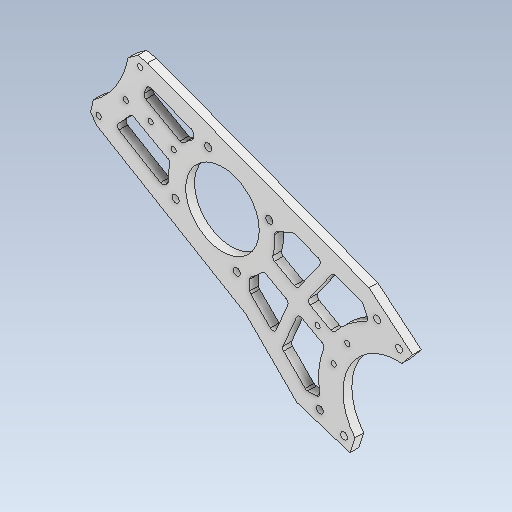
# Autodesk Inventor part: motor_r_1
Saved by Autodesk Inventor 2020 (Build 240168000, 168)
## iProperties
Created: 2020-08-12
Part Number: motor_r_1
Material: ABS Plastic
Document SubType Name: Modeling
Designer: psrobotics
Density: 1.06 g/cm^3
Appearance: Smooth - White
Author: psrobotics
Autodesk Inventor part; units mm, degrees
ref_plane "YZ Plane" through (0, 0, 0) normal (1, 0, 0) x (0, 1, 0)
ref_plane "XZ Plane" through (0, 0, 0) normal (0, 1, 0) x (-1, 0, 0)
ref_plane "XY Plane" through (0, 0, 0) normal (0, 0, 1) x (1, 0, 0)
sketch "Sketch1" plane through (0, 0, 0) normal (0, 0, 1) x (1, 0, 0)
  circle A0 centre (-61.1849, 56.2101) radius 2 projected
  circle A1 centre (-79.1833, 55.9721) radius 2 projected
  circle A2 centre (-87.9764, 40.2661) radius 2 projected
  circle A3 centre (-78.7712, 24.7979) radius 2 projected
  circle A4 centre (-60.7727, 25.0359) radius 2 projected
  circle A5 centre (-51.9796, 40.742) radius 2 projected
  circle A6 centre (39.2427, 1.4435) radius 2.05 projected
  circle A7 centre (33.5273, 15.312) radius 2.05 projected
  circle A8 centre (27.8118, 29.1804) radius 2.05 projected
  line L0 (-22.6947, 30.3679) -> (-27.7397, 36.0115) projected
  arc A9 (-27.2107, 40.4775) -> (-27.7397, 36.0115) centre (-25.5031, 38.0109) ccw projected
  arc A10 (-20.7425, 44.2388) -> (-27.2107, 40.4775) centre (-0.1733, 1.4234) ccw projected
  arc A11 (-16.6578, 42.6485) -> (-20.7425, 44.2388) centre (-19.4434, 41.5346) ccw projected
  line L1 (-16.6578, 42.6485) -> (-13.8655, 35.6655) projected
  arc A12 (-15.3151, 31.8656) -> (-13.8655, 35.6655) centre (-16.6511, 34.5516) ccw projected
  arc A13 (-15.3151, 31.8656) -> (-18.8133, 29.8584) centre (-0.1733, 1.4234) ccw projected
  arc A14 (-22.6947, 30.3679) -> (-18.8133, 29.8584) centre (-20.4581, 32.3673) ccw projected
  line L2 (4.9218, -40.8928) -> (6.6144, -39.5468) projected
  arc A15 (9.7386, -40.4282) -> (6.6144, -39.5468) centre (7.8592, -41.1122) ccw projected
  line L3 (9.7386, -40.4282) -> (10.4367, -42.3462) projected
  arc A16 (8.0919, -44.9753) -> (10.4367, -42.3462) centre (8.5573, -43.0302) ccw projected
  line L4 (8.0919, -44.9753) -> (5.7012, -44.4033) projected
  arc A17 (4.9218, -40.8928) -> (5.7012, -44.4033) centre (6.1666, -42.4582) ccw projected
  line L5 (-46.4911, 13.9051) -> (-45.8812, 17.2926) projected
  arc A18 (-42.9676, 18.7008) -> (-45.8812, 17.2926) centre (-43.9129, 16.9383) ccw projected
  line L6 (-42.9676, 18.7008) -> (-40.9403, 17.6135) projected
  arc A19 (-40.5709, 14.3438) -> (-40.9403, 17.6135) centre (-41.8856, 15.851) ccw projected
  line L7 (-40.5709, 14.3438) -> (-43.208, 12.0435) projected
  arc A20 (-46.4911, 13.9051) -> (-43.208, 12.0435) centre (-44.5227, 13.5507) ccw projected
  arc A21 (20.902, 43.992) -> (13.9559, 46.7733) centre (-0.1733, 1.4234) ccw projected
  arc A22 (22.1637, 39.7941) -> (20.902, 43.992) centre (19.571, 41.3034) ccw projected
  line L8 (22.1637, 39.7941) -> (18.3801, 33.2946) projected
  arc A23 (14.4933, 32.0974) -> (18.3801, 33.2946) centre (15.7874, 34.8039) ccw projected
  arc A24 (14.4933, 32.0974) -> (10.7578, 33.6183) centre (-0.1733, 1.4234) ccw projected
  arc A25 (8.7698, 36.9905) -> (10.7578, 33.6183) centre (11.7223, 36.459) ccw projected
  line L9 (8.7698, 36.9905) -> (10.111, 44.4407) projected
  arc A26 (13.9559, 46.7733) -> (10.111, 44.4407) centre (13.0635, 43.9091) ccw projected
  line L10 (15.012, -40.2978) -> (12.4398, -33.2308) projected
  arc A27 (14.0077, -29.4781) -> (12.4398, -33.2308) centre (15.2589, -32.2047) ccw projected
  arc A28 (14.0077, -29.4781) -> (21.8399, -24.4884) centre (-0.1733, 1.4234) ccw projected
  arc A29 (25.9036, -24.6534) -> (21.8399, -24.4884) centre (23.7822, -26.7747) ccw projected
  line L11 (25.9036, -24.6534) -> (31.2214, -29.9713) projected
  arc A30 (31.0736, -34.3521) -> (31.2214, -29.9713) centre (29.1001, -32.0926) ccw projected
  arc A31 (19.0449, -42.0152) -> (31.0736, -34.3521) centre (-0.1733, 1.4234) ccw projected
  arc A32 (15.012, -40.2978) -> (19.0449, -42.0152) centre (17.8311, -39.2717) ccw projected
  line L12 (-31.4674, 32.6792) -> (-26.4223, 27.0356) projected
  arc A33 (-26.3493, 23.1217) -> (-26.4223, 27.0356) centre (-28.659, 25.0362) ccw projected
  arc A34 (-26.3493, 23.1217) -> (-28.7345, 19.8693) centre (-0.1733, 1.4234) ccw projected
  arc A35 (-32.6725, 18.8531) -> (-28.7345, 19.8693) centre (-31.2547, 21.4969) ccw projected
  line L13 (-32.6725, 18.8531) -> (-39.3001, 22.4076) projected
  arc A36 (-40.4244, 26.6443) -> (-39.3001, 22.4076) centre (-37.8823, 25.0514) ccw projected
  arc A37 (-35.9645, 32.6522) -> (-40.4244, 26.6443) centre (-0.1733, 1.4234) ccw projected
  arc A38 (-31.4674, 32.6792) -> (-35.9645, 32.6522) centre (-33.704, 30.6798) ccw projected
  line L14 (37.0627, -22.7579) -> (30.7554, -18.6619) projected
  arc A39 (29.7491, -14.7214) -> (30.7554, -18.6619) centre (32.3893, -16.1459) ccw projected
  arc A40 (29.7491, -14.7214) -> (31.8466, -10.0103) centre (-0.1733, 1.4234) ccw projected
  arc A41 (35.4483, -8.1214) -> (31.8466, -10.0103) centre (34.6719, -11.0192) ccw projected
  line L15 (35.4483, -8.1214) -> (42.7127, -10.0678) projected
  arc A42 (44.775, -13.9357) -> (42.7127, -10.0678) centre (41.9362, -12.9656) ccw projected
  arc A43 (41.317, -21.7025) -> (44.775, -13.9357) centre (-0.1733, 1.4234) ccw projected
  arc A44 (37.0627, -22.7579) -> (41.317, -21.7025) centre (38.6966, -20.2419) ccw projected
  line L16 (5.1901, 45.3265) -> (3.8489, 37.8764) projected
  arc A45 (0.8096, 35.4092) -> (3.8489, 37.8764) centre (0.8963, 38.4079) ccw projected
  arc A46 (0.8096, 35.4092) -> (-3.2217, 35.2865) centre (-0.1733, 1.4234) ccw projected
  arc A47 (-6.447, 37.764) -> (-3.2217, 35.2865) centre (-3.4907, 38.2744) ccw projected
  line L17 (-6.447, 37.764) -> (-7.7264, 45.175) projected
  arc A48 (-5.08, 48.6693) -> (-7.7264, 45.175) centre (-4.7701, 45.6853) ccw projected
  arc A49 (2.4, 48.8536) -> (-5.08, 48.6693) centre (-0.1733, 1.4234) ccw projected
  arc A50 (5.1901, 45.3265) -> (2.4, 48.8536) centre (2.2375, 45.858) ccw projected
  line L18 (1.7065, -37.0615) -> (-5.4722, -42.7701) projected
  line L19 (-5.4722, -42.7701) -> (-0.1588, -48.8615) projected
  arc A51 (0.3036, -49.8289) -> (-0.1588, -48.8615) centre (-1.666, -50.1762) ccw projected
  line L20 (0.3036, -49.8289) -> (1.5962, -57.1593) projected
  line L21 (1.5962, -57.1593) -> (13.8376, -55.0009) projected
  line L22 (13.8376, -55.0009) -> (13.4343, -52.7138) projected
  arc A52 (14.8476, -50.4454) -> (13.4343, -52.7138) centre (15.4039, -52.3665) ccw projected
  arc A53 (14.8476, -50.4454) -> (24.4955, -46.6125) centre (-0.1733, 1.4234) ccw projected
  arc A54 (27.0802, -47.2926) -> (24.4955, -46.6125) centre (25.4092, -48.3917) ccw projected
  line L23 (27.0802, -47.2926) -> (28.3563, -49.2329) projected
  line L24 (28.3563, -49.2329) -> (35.0402, -44.8369) projected
  line L25 (35.0402, -44.8369) -> (33.7641, -42.8966) projected
  arc A55 (34.1633, -40.2539) -> (33.7641, -42.8966) centre (35.435, -41.7975) ccw projected
  arc A56 (34.1633, -40.2539) -> (41.5041, -32.9132) centre (-0.1733, 1.4234) ccw projected
  arc A57 (44.1467, -32.5139) -> (41.5041, -32.9132) centre (43.0477, -34.1849) ccw projected
  line L26 (44.1467, -32.5139) -> (46.087, -33.7901) projected
  line L27 (46.087, -33.7901) -> (50.4831, -27.1062) projected
  line L28 (50.4831, -27.1062) -> (48.5428, -25.83) projected
  arc A58 (47.8627, -23.2454) -> (48.5428, -25.83) centre (49.6418, -24.159) ccw projected
  arc A59 (47.8627, -23.2454) -> (51.6956, -13.5974) centre (-0.1733, 1.4234) ccw projected
  arc A60 (53.9639, -12.1842) -> (51.6956, -13.5974) centre (53.6166, -14.1538) ccw projected
  line L29 (53.9639, -12.1842) -> (56.251, -12.5874) projected
  line L30 (56.251, -12.5874) -> (57.764, -4.0066) projected
  line L31 (57.764, -4.0066) -> (50.7504, -2.7699) projected
  arc A61 (49.2479, -1.5605) -> (50.7504, -2.7699) centre (51.0977, -0.8002) ccw projected
  line L32 (49.2479, -1.5605) -> (34.2938, 34.8242) projected
  arc A62 (34.7161, 36.9851) -> (34.2938, 34.8242) centre (36.1437, 35.5844) ccw projected
  line L33 (34.7161, 36.9851) -> (37.6444, 39.9698) projected
  line L34 (37.6444, 39.9698) -> (40.1908, 42.9826) projected
  line L35 (40.1908, 42.9826) -> (34.0809, 48.1469) projected
  line L36 (34.0809, 48.1469) -> (33.2883, 47.209) projected
  arc A63 (29.3565, 46.6339) -> (33.2883, 47.209) centre (30.9971, 49.1456) ccw projected
  arc A64 (29.3565, 46.6339) -> (19.0204, 51.8972) centre (-0.1733, 1.4234) ccw projected
  arc A65 (17.5237, 53.1421) -> (19.0204, 51.8972) centre (20.0867, 54.7013) ccw projected
  line L37 (17.5237, 53.1421) -> (1.2772, 56.0668) projected
  arc A66 (-0.5596, 55.422) -> (1.2772, 56.0668) centre (-0.5811, 58.4219) ccw projected
  arc A67 (-0.5596, 55.422) -> (-12.0824, 54.0938) centre (-0.1733, 1.4234) ccw projected
  arc A68 (-15.5667, 56.004) -> (-12.0824, 54.0938) centre (-12.744, 57.0199) ccw projected
  line L38 (-15.5667, 56.004) -> (-15.9826, 57.1593) projected
  line L39 (-15.9826, 57.1593) -> (-66.6416, 64.271) projected
  arc A69 (-66.6416, 64.271) -> (-80.5887, 18.977) centre (-69.978, 40.504) ccw projected
  line L40 (-80.5887, 18.977) -> (-57.764, 7.7267) projected
  line L41 (-57.764, 7.7267) -> (-53.8816, 7.0278) projected
  line L42 (-53.8816, 7.0278) -> (-49.1938, 6.5386) projected
  arc A70 (-47.8942, 5.8641) -> (-49.1938, 6.5386) centre (-49.4014, 4.5494) ccw projected
  line L43 (-47.8942, 5.8641) -> (-45.6437, 3.2841) projected
  line L44 (-45.6437, 3.2841) -> (-37.685, 10.2263) projected
  arc A71 (-31.0721, 6.849) -> (-37.685, 10.2263) centre (-35.0556, 7.2119) ccw projected
  line L45 (-31.0721, 6.849) -> (-32.7441, -11.5046) projected
  line L46 (-32.7441, -11.5046) -> (-18.0587, -28.3404) projected
  line L47 (-18.0587, -28.3404) -> (-0.4203, -29.9472) projected
  arc A72 (1.7065, -37.0615) -> (-0.4203, -29.9472) centre (-0.7832, -33.9307) ccw projected
  line L48 (-19.335, 18.2488) -> (-14.2914, 9.8007) projected
  arc A73 (-15.0846, 8.2903) -> (-14.2914, 9.8007) centre (-15.1501, 9.2881) ccw projected
  line L49 (-15.0846, 8.2903) -> (-24.9026, 7.6464) projected
  arc A74 (-26.4331, 9.5885) -> (-24.9026, 7.6464) centre (-25.0008, 9.1432) ccw projected
  arc A75 (-21.8027, 18.4062) -> (-26.4331, 9.5885) centre (-0.1733, 1.4234) ccw projected
  arc A76 (-19.335, 18.2488) -> (-21.8027, 18.4062) centre (-20.6229, 17.4799) ccw projected
  line L50 (-25.62, -0.2287) -> (-16.08, -2.636) projected
  arc A77 (-15.5728, -4.2649) -> (-16.08, -2.636) centre (-16.3246, -3.6056) ccw projected
  line L51 (-15.5728, -4.2649) -> (-22.0599, -11.6626) projected
  arc A78 (-24.5154, -11.3715) -> (-22.0599, -11.6626) centre (-23.1877, -10.6736) ccw projected
  arc A79 (-27.4763, -1.8623) -> (-24.5154, -11.3715) centre (-0.1733, 1.4234) ccw projected
  arc A80 (-25.62, -0.2287) -> (-27.4763, -1.8623) centre (-25.987, -1.6831) ccw projected
  line L52 (-16.9986, -17.7383) -> (-8.5506, -12.6948) projected
  arc A81 (-7.0401, -13.488) -> (-8.5506, -12.6948) centre (-8.038, -13.5534) ccw projected
  line L53 (-7.0401, -13.488) -> (-6.3962, -23.3059) projected
  arc A82 (-8.3384, -24.8365) -> (-6.3962, -23.3059) centre (-7.893, -23.4041) ccw projected
  arc A83 (-17.1561, -20.2061) -> (-8.3384, -24.8365) centre (-0.1733, 1.4234) ccw projected
  arc A84 (-16.9986, -17.7383) -> (-17.1561, -20.2061) centre (-16.2297, -19.0263) ccw projected
  line L54 (1.4788, -24.0233) -> (3.8861, -14.4833) projected
  arc A85 (5.5151, -13.9761) -> (3.8861, -14.4833) centre (4.8558, -14.728) ccw projected
  line L55 (5.5151, -13.9761) -> (12.9127, -20.4632) projected
  arc A86 (12.6216, -22.9188) -> (12.9127, -20.4632) centre (11.9237, -21.591) ccw projected
  arc A87 (3.1124, -25.8796) -> (12.6216, -22.9188) centre (-0.1733, 1.4234) ccw projected
  arc A88 (1.4788, -24.0233) -> (3.1124, -25.8796) centre (2.9332, -24.3904) ccw projected
  line L56 (18.9885, -15.402) -> (13.9449, -6.9539) projected
  arc A89 (14.7381, -5.4435) -> (13.9449, -6.9539) centre (14.8035, -6.4413) ccw projected
  line L57 (14.7381, -5.4435) -> (24.5561, -4.7996) projected
  arc A90 (26.0866, -6.7418) -> (24.5561, -4.7996) centre (24.6543, -6.2964) ccw projected
  arc A91 (21.4562, -15.5594) -> (26.0866, -6.7418) centre (-0.1733, 1.4234) ccw projected
  arc A92 (18.9885, -15.402) -> (21.4562, -15.5594) centre (20.2764, -14.6331) ccw projected
  line L58 (25.2735, 3.0755) -> (15.7335, 5.4828) projected
  arc A93 (15.2263, 7.1117) -> (15.7335, 5.4828) centre (15.9781, 6.4524) ccw projected
  line L59 (15.2263, 7.1117) -> (21.7134, 14.5094) projected
  arc A94 (24.1689, 14.2183) -> (21.7134, 14.5094) centre (22.8412, 13.5204) ccw projected
  arc A95 (27.1298, 4.7091) -> (24.1689, 14.2183) centre (-0.1733, 1.4234) ccw projected
  arc A96 (25.2735, 3.0755) -> (27.1298, 4.7091) centre (25.6405, 4.5299) ccw projected
  line L60 (16.6521, 20.5851) -> (8.2041, 15.5416) projected
  arc A97 (6.6936, 16.3348) -> (8.2041, 15.5416) centre (7.6915, 16.4002) ccw projected
  line L61 (6.6936, 16.3348) -> (6.0497, 26.1527) projected
  arc A98 (7.9919, 27.6833) -> (6.0497, 26.1527) centre (7.5465, 26.2509) ccw projected
  arc A99 (16.8096, 23.0529) -> (7.9919, 27.6833) centre (-0.1733, 1.4234) ccw projected
  arc A100 (16.6521, 20.5851) -> (16.8096, 23.0529) centre (15.8832, 21.8731) ccw projected
  line L62 (-1.8253, 26.8701) -> (-4.2326, 17.3301) projected
  arc A101 (-5.8616, 16.8229) -> (-4.2326, 17.3301) centre (-5.2023, 17.5748) ccw projected
  line L63 (-5.8616, 16.8229) -> (-13.2592, 23.31) projected
  arc A102 (-12.9681, 25.7656) -> (-13.2592, 23.31) centre (-12.2702, 24.4378) ccw projected
  arc A103 (-3.4589, 28.7264) -> (-12.9681, 25.7656) centre (-0.1733, 1.4234) ccw projected
  arc A104 (-1.8253, 26.8701) -> (-3.4589, 28.7264) centre (-3.2797, 27.2372) ccw projected
  circle A105 centre (10.0674, -10.8701) radius 2 projected
  circle A106 centre (-10.4139, 13.7169) radius 2 projected
  circle A107 centre (-15.1114, 2.7842) radius 1.5 projected
  circle A108 centre (14.7649, 0.0626) radius 1.5 projected
  circle A109 centre (-1.5341, -13.5147) radius 1.5 projected
  circle A110 centre (1.1876, 16.3615) radius 1.5 projected
  circle A111 centre (-12.4667, -8.8173) radius 2 projected
  circle A112 centre (12.1202, 11.664) radius 2 projected
  circle A113 centre (-0.1733, 1.4234) radius 12 projected
  circle A114 centre (-18.3916, 52.0411) radius 1.55 projected
  circle A115 centre (53.4988, -8.0404) radius 1.55 projected
  circle A116 centre (29.775, -44.1107) radius 1.55 projected
  circle A117 centre (9.2906, -52.2486) radius 1.55 projected
  circle A118 centre (45.3608, -28.5248) radius 1.55 projected
  circle A119 centre (34.5538, 42.5098) radius 1.55 projected
  circle A120 centre (-53.1186, 10.9547) radius 1.55 projected
  circle A121 centre (200.5155, -110.9334) radius 35 projected
  line L64 (28.3563, -49.2329) -> (182.6199, -141.0124)
  line L65 (57.764, -4.0066) -> (215.5932, -79.3476)
  circle A122 centre (-0.1733, 1.4234) radius 47.5
  line L66 (28.3563, -49.2329) -> (22.4938, -40.3193)
  line L67 (57.764, -4.0066) -> (47.1927, -2.1425)
  point P0 (0, 0)
  point P1 (44.775, -13.9357)
  point P2 (41.317, -21.7025)
  constraints: 8 end point, 4 point on circle, 2 collinear, 2 tangent, 1 centre point, 1 coincident, 1 concentric
extrude "Extrusion1" add sketch "Sketch1" along normal blind 5 contours A31 A122 A43 L67 L31 L30 L29 A60 A59 A58 L28 L27 L26 A57 A56 A55 L25 L24 L23 L66 | L65 A121 L64 L24 L25 A55 A56 A57 L26 L27 L28 A58 A59 A60 L29 L30
sketch "Sketch2" plane through (0, 0, 5) normal (0, 0, 1) x (1, 0, 0)
  circle A0 centre (100.6074, -54.9992) radius 17.5 projected
  circle A1 centre (100.6074, -54.9992) radius 21
  point P0 (0, 0)
  dimension "d5" = 42
  constraints: 1 centre point, 1 coincident
  measures "d5" diameter of A1
extrude "Extrusion2" cut sketch "Sketch2" against normal blind 5 contours A0 | A1
sketch "Sketch3" plane through (0, 0, 5) normal (0, 0, 1) x (1, 0, 0)
  circle A0 centre (156.3377, -126.3623) radius 2 projected
  circle A1 centre (170.0821, -132.37) radius 2 projected
  line L0 (189.8622, -144.2727) -> (191.6885, -138.5574) projected
  arc A2 (185.6877, -135.856) -> (191.6885, -138.5574) centre (200.5155, -110.9334) ccw projected
  line L1 (151.3117, -115.4039) -> (185.6877, -135.856) projected
  line L2 (143.0379, -129.3104) -> (151.3117, -115.4039) projected
  line L3 (189.8622, -144.2727) -> (143.0379, -129.3104) projected
  circle A3 centre (201.5033, -73.4985) radius 2 projected
  circle A4 centre (188.9781, -65.2451) radius 2 projected
  line L4 (184.3455, -51.955) -> (222.8987, -84.0263) projected
  line L5 (176.9104, -67.5306) -> (184.3455, -51.955) projected
  line L6 (213.0084, -84.7623) -> (176.9104, -67.5306) projected
  arc A5 (219.0616, -88.6389) -> (213.0084, -84.7623) centre (200.5155, -110.9334) ccw projected
  line L7 (219.0616, -88.6389) -> (222.8987, -84.0263) projected
  arc A6 (215.5932, -79.3476) -> (182.6199, -141.0124) centre (200.5155, -110.9334) ccw projected
  line L8 (200.5155, -110.9334) -> (182.1469, -141.8073)
  line L9 (200.5155, -110.9334) -> (216.071, -78.3466)
  point P0 (0, 0)
  constraints: 4 end point, 4 point on line
extrude "Extrusion3" add sketch "Sketch3" against normal blind 5 contours A0 | A1 | L3 L2 L1 A6 L8 | L8 A6 L1 | A6 L9 L6 | L6 L5 L4 L9 A6 | A3 | A4
thicken "Thicken1" operation add thickness 4 both sides no extend neighbours yes toward (0.637995, -0.7700405, 0) faces at (178.1856, -83.982, 3.3333)
sketch "Sketch4" plane through (0, 0, 5) normal (0, 0, 1) x (1, 0, 0)
  circle A0 centre (53.4988, -8.0404) radius 1.55 projected
  circle A1 centre (29.775, -44.1107) radius 1.55 projected
  circle A2 centre (45.3608, -28.5248) radius 1.55 projected
  circle A3 centre (100.6074, -54.9992) radius 21 projected
  line L0 (213.0084, -84.7623) -> (216.071, -78.3466) projected
  line L1 (216.071, -78.3466) -> (184.3455, -51.955) projected
  line L2 (184.3455, -51.955) -> (179.4951, -62.1159) projected
  line L3 (179.4951, -62.1159) -> (57.764, -4.0066) projected
  line L4 (57.764, -4.0066) -> (47.1927, -2.1425) projected
  arc A4 (22.4938, -40.3193) -> (47.1927, -2.1425) centre (-0.1733, 1.4234) ccw projected
  line L5 (22.4938, -40.3193) -> (28.3563, -49.2329) projected
  line L6 (28.3563, -49.2329) -> (148.2438, -120.5603) projected
  line L7 (148.2438, -120.5603) -> (143.0379, -129.3104) projected
  line L8 (143.0379, -129.3104) -> (182.1469, -141.8073) projected
  line L9 (182.1469, -141.8073) -> (185.6877, -135.856) projected
  line L10 (185.6877, -135.856) -> (176.2734, -130.255) projected
  arc A5 (203.1226, -80.0432) -> (176.2734, -130.255) centre (200.5155, -110.9334) ccw projected
  line L11 (203.1226, -80.0432) -> (213.0084, -84.7623) projected
  line L12 (179.4951, -62.1159) -> (57.764, -4.0066) projected
  line L13 (148.2438, -120.5603) -> (143.0379, -129.3104) projected
  line L14 (148.2438, -120.5603) -> (113.8678, -100.1082)
  line L15 (28.3563, -49.2329) -> (148.2438, -120.5603) projected
  line L16 (143.0379, -129.3104) -> (182.1469, -141.8073) projected
  line L17 (113.8678, -100.1082) -> (143.0379, -129.3104)
  line L18 (184.3455, -51.955) -> (57.764, -4.0066)
  point P0 (0, 0)
  dimension "d13" = 40
  constraints: 6 end point, 1 point on line
  measures "d13" distance of L6.end L14.end
extrude "Extrusion4" add sketch "Sketch4" against normal blind 5 contours L2 L3 L18 | L17 L6 L7
sketch "Sketch5" plane through (0, 0, 5) normal (0, 0, 1) x (1, 0, 0)
  circle A0 centre (188.9781, -65.2451) radius 2 projected
  circle A1 centre (201.5033, -73.4985) radius 2 projected
  circle A2 centre (156.3377, -126.3623) radius 2 projected
  circle A3 centre (170.0821, -132.37) radius 2 projected
  point P0 (0, 0)
extrude "Extrusion5" cut sketch "Sketch5" against normal blind 10
sketch "Sketch6" plane through (0, 0, 0) normal (0, 0, -1) x (-1, 0, 0)
  circle A0 centre (-156.3377, -126.3623) radius 2 projected
  circle A1 centre (-201.5033, -73.4985) radius 2 projected
  circle A2 centre (-170.0821, -132.37) radius 2 projected
  circle A3 centre (-188.9781, -65.2451) radius 2 projected
  arc A4 (-176.2734, -130.255) -> (-203.1226, -80.0432) centre (-200.5155, -110.9334) ccw projected
  line L0 (-176.2734, -130.255) -> (-185.6877, -135.856) projected
  line L1 (-185.6877, -135.856) -> (-182.1469, -141.8073) projected
  line L2 (-182.1469, -141.8073) -> (-143.0379, -129.3104) projected
  line L3 (-143.0379, -129.3104) -> (-113.8678, -100.1082) projected
  line L4 (-28.3563, -49.2329) -> (-113.8678, -100.1082) projected
  line L5 (-22.4938, -40.3193) -> (-28.3563, -49.2329) projected
  arc A5 (-47.1927, -2.1425) -> (-22.4938, -40.3193) centre (0.1733, 1.4234) ccw projected
  line L6 (-57.764, -4.0066) -> (-47.1927, -2.1425) projected
  line L7 (-57.764, -4.0066) -> (-184.3455, -51.955) projected
  line L8 (-184.3455, -51.955) -> (-216.071, -78.3466) projected
  line L9 (-216.071, -78.3466) -> (-213.0084, -84.7623) projected
  line L10 (-213.0084, -84.7623) -> (-203.1226, -80.0432) projected
  circle A6 centre (-100.6074, -54.9992) radius 21 projected
  circle A7 centre (-45.3608, -28.5248) radius 1.55 projected
  circle A8 centre (-29.775, -44.1107) radius 1.55 projected
  circle A9 centre (-53.4988, -8.0404) radius 1.55 projected
  arc A10 (-176.2734, -130.255) -> (-203.1226, -80.0432) centre (-200.5155, -110.9334) ccw projected
  line L11 (-203.1226, -80.0432) -> (-209.2525, -72.6744)
  line L12 (-216.071, -78.3466) -> (-184.3455, -51.955) projected
  line L13 (-176.2734, -130.255) -> (-173.4681, -139.0341)
  line L14 (-143.0379, -129.3104) -> (-182.1469, -141.8073) projected
  point P0 (0, 0)
  constraints: 4 end point, 2 perpendicular, 2 point on line
extrude "Extrusion6" cut sketch "Sketch6" against normal blind 10 contours L13 L2 L1 L0 | L10 L9 L8 L11
sketch "Sketch7" plane through (0, 0, 5) normal (0, 0, 1) x (1, 0, 0)
  circle A0 centre (171.9207, -85.756) radius 2.05 projected
  circle A1 centre (164.1045, -99.7169) radius 2.05 projected
  circle A2 centre (154.9242, -85.4088) radius 2.05 projected
  circle A3 centre (72.6855, -39.367) radius 2.05 projected
  circle A4 centre (59.5971, -32.0394) radius 2.05 projected
  point P0 (0, 0)
hole "Hole1" at (59.5971, -32.0394, 5) at (72.6855, -39.367, 5) at (154.9242, -85.4088, 5) at (171.9207, -85.756, 5) at (164.1045, -99.7169, 5) direction (0, 0, -1) diameter 3 depth 8
sketch "Sketch8" plane through (0, 0, 5) normal (0, 0, 1) x (1, 0, 0)
  circle A0 centre (100.6074, -54.9992) radius 21 projected
  circle A1 centre (72.6855, -39.367) radius 1.5 projected
  circle A2 centre (72.6855, -39.367) radius 1.5 projected
  line L0 (100.6074, -54.9992) -> (72.6855, -39.367)
  line L1 (100.6074, -54.9992) -> (92.421, -28.2227)
  line L2 (100.6074, -54.9992) -> (128.6074, -54.9992) construction
  circle A3 centre (92.421, -28.2227) radius 2.05
  circle A4 centre (73.8308, -63.1856) radius 2.05
  circle A5 centre (108.7938, -81.7758) radius 2.05
  circle A6 centre (127.3839, -46.8128) radius 2.05
  point P0 (0, 0)
  dimension "d27" = 28
  dimension "d28" = 107
  dimension "d29" = 4.1
  dimension "d32" = 360
  constraints: 6 end point, 4 centre point, 1 coincident, 1 equal length, 1 horizontal, 9 other
  measures "d27" distance of L0.start L1.end
  measures "d28" angle of L2 L1
  measures "d29" diameter of A3
extrude "Extrusion7" cut sketch "Sketch8" against normal blind 10 contours A3 | A4 | A5 | A6
sketch "Sketch9" plane through (0, 0, 5) normal (0, 0, 1) x (1, 0, 0)
  arc A0 (203.1226, -80.0432) -> (176.2734, -130.255) centre (200.5155, -110.9334) ccw projected
  circle A1 centre (200.5155, -110.9334) radius 45
  circle A2 centre (100.6074, -54.9992) radius 21 projected
  circle A3 centre (100.6074, -54.9992) radius 30
  line L0 (100.6074, -54.9992) -> (200.5155, -110.9334)
  line L1 (100.6074, -54.9992) -> (200.5155, -110.9334) construction
  line L2 (97.1878, -61.1072) -> (197.0959, -117.0413)
  line L3 (203.935, -104.8255) -> (104.0269, -48.8913)
  arc A4 (104.0269, -48.8913) -> (97.1878, -61.1072) centre (100.6074, -54.9992) ccw
  arc A5 (197.0959, -117.0413) -> (203.935, -104.8255) centre (200.5155, -110.9334) ccw
  line L4 (113.8678, -100.1082) -> (143.0379, -129.3104) projected
  line L5 (111.0396, -83.127) -> (161.9072, -134.0505)
  line L6 (184.3455, -51.955) -> (57.764, -4.0066) projected
  line L7 (127.1273, -40.9744) -> (194.1952, -66.3794)
  line L8 (180.8032, -61.3066) -> (184.2573, -68.973)
  line L9 (148.4428, -120.5713) -> (156.5607, -120.5757)
  line L10 (130.3492, -51.0716) -> (141.0527, -46.2493)
  line L11 (116.2637, -80.5899) -> (116.2594, -88.3525)
  point P0 (0, 0)
  point P1 (150.5614, -82.9663)
  point P2 (158.3087, -95.326)
  point P3 (122.6421, -75.3579)
  point P4 (129.4812, -63.142)
  point P5 (165.1478, -83.1102)
  dimension "d36" = 90
  dimension "d37" = 60
  dimension "d38" = 14
  dimension "d39" = 10
  dimension "d40" = 10
  dimension "d43" = 45
  dimension "d44" = 45
  dimension "d45" = 45
  dimension "d46" = 45
  constraints: 22 end point, 12 point on circle, 4 centre point, 4 point on line, 4 tangent, 3 parallel, 2 coincident, 1 collinear, 1 midpoint
  measures "d36" diameter of A1
  measures "d37" diameter of A3
  measures "d38" diameter of A5
  measures "d39" distance between parallel lines of L4 L5
  measures "d40" distance between parallel lines of L6 L7
  measures "d43" angle of L7 L10
  measures "d44" angle of L5 L11
  measures "d45" angle of L7 L8
  measures "d46" angle of L5 L9
extrude "Extrusion9" cut sketch "Sketch9" against normal blind 10 contours L3 A3 L10 L7 L8 A1 | A1 L9 L5 L11 A3 L2
sketch "Sketch10" plane through (0, 0, 5) normal (0, 0, 1) x (1, 0, 0)
  line L0 (165.1478, -83.1102) -> (129.4812, -63.142) projected
  arc A0 (129.4812, -63.142) -> (130.3492, -51.0716) centre (100.6074, -54.9992) ccw projected
  line L1 (130.3492, -51.0716) -> (141.0527, -46.2493) projected
  line L2 (141.0527, -46.2493) -> (180.8032, -61.3066) projected
  line L3 (180.8032, -61.3066) -> (184.2573, -68.973) projected
  arc A1 (184.2573, -68.973) -> (165.1478, -83.1102) centre (200.5155, -110.9334) ccw projected
  line L4 (122.6421, -75.3579) -> (158.3087, -95.326) projected
  arc A2 (158.3087, -95.326) -> (156.5607, -120.5757) centre (200.5155, -110.9334) ccw projected
  line L5 (156.5607, -120.5757) -> (148.4428, -120.5713) projected
  line L6 (148.4428, -120.5713) -> (116.2594, -88.3525) projected
  line L7 (116.2594, -88.3525) -> (116.2637, -80.5899) projected
  arc A3 (116.2637, -80.5899) -> (122.6421, -75.3579) centre (100.6074, -54.9992) ccw projected
  circle A4 centre (127.3839, -46.8128) radius 2.05 projected
  circle A5 centre (92.421, -28.2227) radius 2.05 projected
  circle A6 centre (108.7938, -81.7758) radius 2.05 projected
  circle A7 centre (73.8308, -63.1856) radius 2.05 projected
  circle A8 centre (171.9207, -85.756) radius 1.5 projected
  circle A9 centre (72.6855, -39.367) radius 1.5 projected
  circle A10 centre (59.5971, -32.0394) radius 1.5 projected
  circle A11 centre (154.9242, -85.4088) radius 1.5 projected
  circle A12 centre (164.1045, -99.7169) radius 1.5 projected
  circle A13 centre (100.6074, -54.9992) radius 21 projected
  circle A14 centre (45.3608, -28.5248) radius 1.55 projected
  circle A15 centre (29.775, -44.1107) radius 1.55 projected
  circle A16 centre (53.4988, -8.0404) radius 1.55 projected
  circle A17 centre (188.9781, -65.2451) radius 2 projected
  circle A18 centre (170.0821, -132.37) radius 2 projected
  circle A19 centre (201.5033, -73.4985) radius 2 projected
  circle A20 centre (156.3377, -126.3623) radius 2 projected
  line L8 (173.4681, -139.0341) -> (176.2734, -130.255) projected
  arc A21 (203.1226, -80.0432) -> (176.2734, -130.255) centre (200.5155, -110.9334) ccw projected
  line L9 (203.1226, -80.0432) -> (209.2525, -72.6744) projected
  line L10 (209.2525, -72.6744) -> (184.3455, -51.955) projected
  line L11 (184.3455, -51.955) -> (57.764, -4.0066) projected
  line L12 (57.764, -4.0066) -> (47.1927, -2.1425) projected
  arc A22 (22.4938, -40.3193) -> (47.1927, -2.1425) centre (-0.1733, 1.4234) ccw projected
  line L13 (22.4938, -40.3193) -> (28.3563, -49.2329) projected
  line L14 (28.3563, -49.2329) -> (113.8678, -100.1082) projected
  line L15 (113.8678, -100.1082) -> (143.0379, -129.3104) projected
  line L16 (143.0379, -129.3104) -> (173.4681, -139.0341) projected
  circle A23 centre (100.6074, -54.9992) radius 31
  circle A24 centre (-0.1733, 1.4234) radius 60
  line L17 (100.6074, -54.9992) -> (-0.1733, 1.4234) construction
  line L18 (104.0269, -48.8913) -> (3.2463, 7.5313)
  line L19 (-3.5928, -4.6845) -> (97.1878, -61.1072)
  arc A25 (97.1878, -61.1072) -> (104.0269, -48.8913) centre (100.6074, -54.9992) ccw
  arc A26 (3.2463, 7.5313) -> (-3.5928, -4.6845) centre (-0.1733, 1.4234) ccw
  line L20 (88.6485, -26.3988) -> (57.6336, -14.6505)
  line L21 (39.0648, -43.968) -> (70.5844, -62.7206)
  line L22 (184.3455, -51.955) -> (57.764, -4.0066) projected
  point P0 (0, 0)
  point P1 (50.2171, -26.7879)
  point P2 (55.2424, -21.579)
  point P3 (77.6762, -34.1387)
  point P4 (70.8371, -46.3545)
  point P5 (48.4033, -33.7948)
  dimension "d49" = 62
  dimension "d50" = 120
  dimension "d51" = 14
  dimension "d52" = 10
  dimension "d53" = 10
  constraints: 12 end point, 8 point on circle, 4 centre point, 4 tangent, 3 parallel, 2 coincident, 1 midpoint
  measures "d49" diameter of A23
  measures "d50" diameter of A24
  measures "d51" diameter of A26
  measures "d52" distance between parallel lines of L11 L20
  measures "d53" distance between parallel lines of L14 L21
extrude "Extrusion10" cut sketch "Sketch10" against normal blind 10 contours L21 A24 L19 A23 | A23 L18 A24 L20
chamfer "Chamfer1" distance 5 angle 45 2 edges at (70.5844, -62.7206, 2.5) (88.6485, -26.3988, 2.5)
sketch "Sketch11" plane through (0, 0, 5) normal (0, 0, 1) x (1, 0, 0)
  line L0 (122.6421, -75.3579) -> (158.3087, -95.326) projected
  line L1 (148.4428, -120.5713) -> (116.2594, -88.3525) projected
  line L2 (165.1478, -83.1102) -> (129.4812, -63.142) projected
  line L3 (141.0527, -46.2493) -> (180.8032, -61.3066) projected
  line L4 (140.4754, -85.3419) -> (132.3511, -104.4619)
  line L5 (116.2594, -88.3525) -> (148.4428, -120.5713) projected
  line L6 (130.0643, -102.1726) -> (137.8422, -83.8677)
  line L7 (143.1086, -86.8162) -> (134.6379, -106.7512)
  line L8 (129.4812, -63.142) -> (165.1478, -83.1102) projected
  line L9 (147.3145, -73.1261) -> (160.9279, -53.7779)
  line L10 (180.8032, -61.3066) -> (141.0527, -46.2493) projected
  line L11 (157.6711, -52.5442) -> (144.3553, -71.4694)
  line L12 (163.8242, -54.875) -> (149.946, -74.5994)
  point P0 (0, 0)
  dimension "d59" = 3
  dimension "d60" = 3
  dimension "d61" = 3
  constraints: 12 end point, 9 point on line, 4 midpoint, 4 parallel
  measures "d59" distance between parallel lines of L4 L7
  measures "d60" distance between parallel lines of L4 L6
  measures "d61" distance between parallel lines of L9 L12
extrude "Extrusion11" add sketch "Sketch11" against normal blind 5
thicken "Thicken2" operation add thickness 2 both sides no extend neighbours yes toward (-0.4885077, -0.8725596, 0) faces at (155.0133, -77.4363, 3.3333) (134.4392, -65.9178, 1.6667)
thicken "Thicken3" operation add thickness 2 both sides no extend neighbours yes toward (0.4885077, 0.8725596, 0) faces at (127.7088, -78.1945, 1.6667) (153.242, -92.4894, 3.3333)
fillet "Fillet4" radius 2 30 edges at (57.6336, -14.6505, 2.5) (55.2424, -21.579, 2.5) (77.6762, -34.1387, 2.5) (84.2061, -28.6934, 2.5) (83.9727, -24.6276, 2.5) (70.8371, -46.3545, 2.5) (48.4033, -33.7948, 2.5) (39.0648, -43.968, 2.5) (66.2874, -60.1641, 2.5) (69.7336, -57.7935, 2.5) (130.3492, -51.0716, 2.5) (141.0527, -46.2493, 2.5) (157.6711, -52.5442, 2.5) (143.1983, -73.1137, 2.5) (128.8606, -65.0867, 2.5) (148.7891, -76.2438, 2.5) (163.8242, -54.875, 2.5) (180.8032, -61.3066, 2.5) (184.2573, -68.973, 2.5) (163.9359, -84.7238, 2.5) (159.0509, -93.4494, 2.5) (143.8953, -84.9645, 2.5) (134.6379, -106.7512, 2.5) (148.4428, -120.5713, 2.5) (156.5607, -120.5757, 2.5) (130.0643, -102.1726, 2.5) (138.629, -82.0161, 2.5) (123.9755, -73.8123, 2.5) (116.2637, -80.5899, 2.5) (116.2594, -88.3525, 2.5)
chamfer "Chamfer2" distance 5 angle 45 2 edges at (47.1927, -2.1425, 2.5) (22.4938, -40.3193, 2.5)
body "Solid1"
